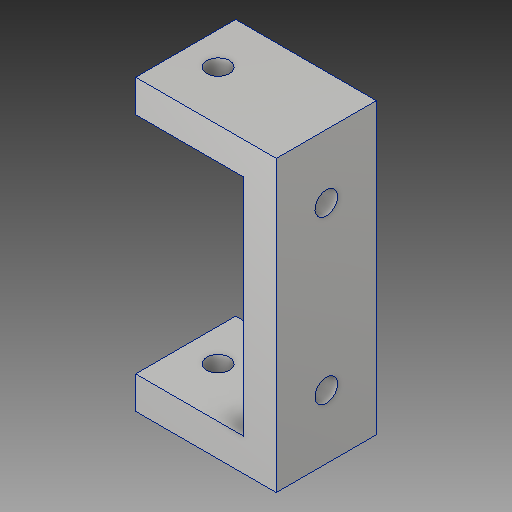
# Autodesk Inventor part: End Bracing
Saved by Autodesk Inventor 2019.4 (Build 234330000, 330)
## iProperties
Created: 2019-12-14
Part Number: End Bracing
Material: Aluminum 6061
Document SubType Name: Modeling
Designer: Mark
Mass: 27.1242 g
Surface Area: 50.0934 cm^2
Volume: 10.046 cm^3
Density: 2.7 g/cm^3
Appearance: Aluminum - Flat
Author: Mark
Autodesk Inventor part; units mm, degrees
ref_plane "YZ Plane" through (0, 0, 0) normal (1, 0, 0) x (0, 1, 0)
ref_plane "XZ Plane" through (0, 0, 0) normal (0, 1, 0) x (-1, 0, 0)
ref_plane "XY Plane" through (0, 0, 0) normal (0, 0, 1) x (1, 0, 0)
sketch "Sketch1" plane through (0, 0, 0) normal (1, 0, 0) x (0, 1, 0)
  line L0 (-26.75, 9.25) -> (26.75, 9.25)
  line L1 (26.75, 9.25) -> (26.75, -9.25)
  line L2 (26.75, -9.25) -> (-26.75, -9.25)
  line L3 (-26.75, -9.25) -> (-26.75, 9.25)
  line L4 (-26.75, 9.25) -> (26.75, -9.25) construction
  line L5 (26.75, 9.25) -> (-26.75, -9.25) construction
  circle A0 centre (15, 0) radius 2.1
  circle A1 centre (-15, 0) radius 2.1
  point P0 (0, 0)
  dimension "d0" = 53.5
  dimension "d1" = 18.5
  dimension "d2" = 4.2
  dimension "d3" = 4.2
  dimension "d4" = 30
  dimension "d5" = 11.75
  dimension "d6" = 9.25
  dimension "d7" = 9.25
  constraints: 12 end point, 2 centre point, 2 midpoint, 2 parallel, 1 horizontal, 1 perpendicular
  measures "d0" distance of L1.end L2.end
  measures "d1" distance of L0.end L1.end
  measures "d2" diameter of A0
  measures "d3" diameter of A1
  measures "d4" distance of A1.centre A0.centre
  measures "d5" distance from line of L1 A0.centre
  measures "d6" distance from line of L2 A0.centre
  measures "d7" distance from line of L2 A1.centre
extrude "Extrusion1" add sketch "Sketch1" along normal blind 6
sketch "Sketch2" plane through (0, 0, 0) normal (-1, 0, 0) x (0, 0, 1)
  line L0 (-9.25, 26.75) -> (9.25, 26.75) projected
  line L1 (-9.25, 26.75) -> (9.25, 26.75)
  line L2 (9.25, 26.75) -> (9.25, 20.75)
  line L3 (9.25, 20.75) -> (-9.25, 20.75)
  line L4 (-9.25, 20.75) -> (-9.25, 26.75)
  line L5 (9.25, 26.75) -> (9.25, -26.75) projected
  line L6 (9.25, -26.75) -> (-9.25, -26.75)
  line L7 (-9.25, -26.75) -> (-9.25, -20.75)
  line L8 (-9.25, -20.75) -> (9.25, -20.75)
  line L9 (9.25, -20.75) -> (9.25, -26.75)
  point P0 (0, 0)
  dimension "d10" = 18.5
  dimension "d11" = 6
  dimension "d12" = 18.5
  dimension "d13" = 6
  constraints: 16 end point, 4 parallel, 2 horizontal, 2 perpendicular
  measures "d10" distance of L2.end L3.end
  measures "d11" distance of L1.end L2.end
  measures "d12" distance of L7.end L8.end
  measures "d13" distance of L6.end L7.end
extrude "Extrusion2" add sketch "Sketch2" along normal blind 20
sketch "Sketch3" plane through (6, 26.75, 9.25) normal (0, 1, 0) x (1, 0, 0)
  circle A0 centre (-20, 9.25) radius 2.1
  line L0 (0, 0) -> (-26, 0) projected
  line L1 (0, 18.5) -> (0, 0) projected
  point P0 (-6, 9.25)
  dimension "d16" = 4.2
  dimension "d18" = 20
  dimension "d21" = 9.25
  constraints: 1 centre point
  measures "d16" diameter of A0
  measures "d18" distance from line of L1 A0.centre
  measures "d21" distance from line of L0 A0.centre
extrude "Extrusion3" cut sketch "Sketch3" against normal blind 100
equation "\"d7\" = d6"
body "Solid1"
